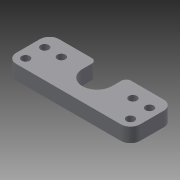
# Autodesk Inventor part: Extruder_Fixer_normal
Saved by Autodesk Inventor 2014 (Build 180170000, 170)
## iProperties
Created: 2015-12-28
Part Number: Extruder_Fixer_normal
Material: Generic
Document SubType Name: Modeling
Designer: inornate
Density: 1 g/cm^3
Appearance: Default
Author: inornate
Autodesk Inventor part; units mm, degrees
ref_plane "YZ Plane" through (0, 0, 0) normal (1, 0, 0) x (0, 1, 0)
ref_plane "XZ Plane" through (0, 0, 0) normal (0, 1, 0) x (-1, 0, 0)
ref_plane "XY Plane" through (0, 0, 0) normal (0, 0, 1) x (1, 0, 0)
sketch "Sketch1" plane through (0, 0, 0) normal (0, 0, 1) x (1, 0, 0)
  circle A0 centre (18.6957, -1.4966) radius 1.7
  circle A1 centre (18.6957, 6.5034) radius 1.7 projected
  circle A2 centre (11.6957, 6.5034) radius 1.7 projected
  arc A3 (22.6957, 8.5034) -> (18.6957, 12.5034) centre (18.6957, 8.5034) ccw
  line L0 (4.8957, 12.5034) -> (18.6957, 12.5034)
  arc A4 (4.8957, 12.5034) -> (2.8957, 10.5034) centre (4.8957, 10.5034) ccw
  line L1 (2.8957, 6.5034) -> (2.8957, 10.5034)
  arc A5 (-9.5043, 6.5034) -> (2.8957, 6.5034) centre (-3.3043, 6.5034) ccw projected
  line L2 (-9.5043, 10.5034) -> (-9.5043, 6.5034)
  arc A6 (-9.5043, 10.5034) -> (-11.5043, 12.5034) centre (-11.5043, 10.5034) ccw
  line L3 (22.6957, 8.5034) -> (22.6957, -1.4966)
  arc A7 (18.6957, -5.4966) -> (22.6957, -1.4966) centre (18.6957, -1.4966) ccw
  line L4 (-3.3043, 6.5034) -> (-3.3043, -12.8188) construction
  circle A8 centre (-25.3043, -1.4966) radius 1.7
  circle A9 centre (-25.3043, 6.5034) radius 1.7
  circle A10 centre (-18.3043, 6.5034) radius 1.7
  arc A11 (-25.3043, 12.5034) -> (-29.3043, 8.5034) centre (-25.3043, 8.5034) ccw
  line L5 (-11.5043, 12.5034) -> (-25.3043, 12.5034)
  line L6 (-9.5043, 6.5034) -> (-9.5043, 10.5034)
  arc A12 (-9.5043, 6.5034) -> (2.8957, 6.5034) centre (-3.3043, 6.5034) ccw
  line L7 (-29.3043, 8.5034) -> (-29.3043, -1.4966)
  arc A13 (-29.3043, -1.4966) -> (-25.3043, -5.4966) centre (-25.3043, -1.4966) ccw
  line L8 (-25.3043, -5.4966) -> (18.6957, -5.4966)
  point P0 (0, 0)
  dimension "d18" = 4
  dimension "d24" = 6
  dimension "d26" = 2
  dimension "d27" = 2
  dimension "d28" = 2
  constraints: 18 end point, 14 point on circle, 11 centre point, 11 symmetric about line, 3 tangent, 2 parallel, 1 horizontal, 1 horizontal alignment, 1 perpendicular, 1 vertical alignment, 6 other
  measures "d18" radius of A7
  measures "d24" distance from line of L0 L4.start
  measures "d26" distance from line of L2 A6.centre
  measures "d27" radius of A4
  measures "d28" distance from line of A4.centre L1
extrude "Extrusion1" add sketch "Sketch1" against normal blind 6
sketch "Sketch2" plane through (0, 0, -6) normal (0, 0, -1) x (-1, 0, 0)
  circle A0 centre (26.3043, -2.4966) radius 1.6 projected
  circle A1 centre (26.3043, 15.5034) radius 1.6 projected
  circle A2 centre (26.3043, 6.5034) radius 2.5 projected
  arc A3 (30.3043, 15.5034) -> (23.3147, 18.1609) centre (26.3043, 15.5034) ccw projected
  circle A4 centre (18.3043, 6.5034) radius 1.7 projected
  circle A5 centre (18.3043, -5.4966) radius 1.7 projected
  circle A6 centre (26.3043, -2.4966) radius 1.6 projected
  circle A7 centre (26.3043, 15.5034) radius 1.6 projected
  line L0 (14.3043, 6.5034) -> (14.3043, -5.4966) projected
  arc A8 (14.3043, -5.4966) -> (19.7088, -9.2419) centre (18.3043, -5.4966) ccw projected
  line L1 (19.7088, -9.2419) -> (27.7088, -6.2419) projected
  arc A9 (27.7088, -6.2419) -> (30.3043, -2.4966) centre (26.3043, -2.4966) ccw projected
  line L2 (30.3043, -2.4966) -> (30.3043, 2.0313) projected
  arc A10 (30.3043, 2.0313) -> (30.3043, 10.9756) centre (26.3043, 6.5034) ccw projected
  line L3 (30.3043, 10.9756) -> (30.3043, 15.5034) projected
  arc A11 (30.3043, 15.5034) -> (23.3147, 18.1609) centre (26.3043, 15.5034) ccw projected
  line L4 (23.3147, 18.1609) -> (15.3147, 9.1609) projected
  arc A12 (15.3147, 9.1609) -> (14.3043, 6.5034) centre (18.3043, 6.5034) ccw projected
  line L5 (18.3043, 12.5242) -> (23.3147, 18.1609) construction
  arc A13 (27.7088, -6.2419) -> (18.3043, -5.4966) centre (19.7185, -47.358) ccw projected
  line L6 (23.3147, 18.1609) -> (16.508, 12.5034) projected
  line L7 (-4.8957, 12.5034) -> (-18.6957, 12.5034) projected
  line L8 (21.8043, 16.9055) -> (21.8043, -5.5246)
  line L9 (25.163, -7.1966) -> (21.8043, -5.5246)
  circle A14 centre (18.3043, 6.5034) radius 1.7 projected
  point P0 (0, 0)
  dimension "d22" = 3.5
  constraints: 6 end point, 2 point on line, 2 tangent, 1 coincident, 1 perpendicular, 1 point on circle, 3 other
  measures "d22" distance from line of L8 A14.centre
sketch "Sketch4" plane through (0, 0, -6) normal (0, 0, -1) x (-1, 0, 0)
  circle A0 centre (-11.6957, 6.5034) radius 1.7 projected
  circle A1 centre (18.3043, 6.5034) radius 1.7 projected
  line L0 (-8.4337, 6.5034) -> (-10.0647, 3.6784)
  line L1 (-10.0647, 3.6784) -> (-13.3267, 3.6784)
  line L2 (-13.3267, 3.6784) -> (-14.9577, 6.5034)
  line L3 (-14.9577, 6.5034) -> (-13.3267, 9.3284)
  line L4 (-13.3267, 9.3284) -> (-10.0647, 9.3284)
  line L5 (-10.0647, 9.3284) -> (-8.4337, 6.5034)
  line L6 (15.0423, 6.5034) -> (16.6733, 9.3284)
  line L7 (16.6733, 9.3284) -> (19.9353, 9.3284)
  line L8 (19.9353, 9.3284) -> (21.5663, 6.5034)
  line L9 (21.5663, 6.5034) -> (19.9353, 3.6784)
  line L10 (19.9353, 3.6784) -> (16.6733, 3.6784)
  line L11 (16.6733, 3.6784) -> (15.0423, 6.5034)
  dimension "d21" = 5.65
  constraints: 24 end point, 2 coincident, 1 collinear, 26 other
  measures "d21" distance between parallel lines of L1 L4
body "Solid1"
